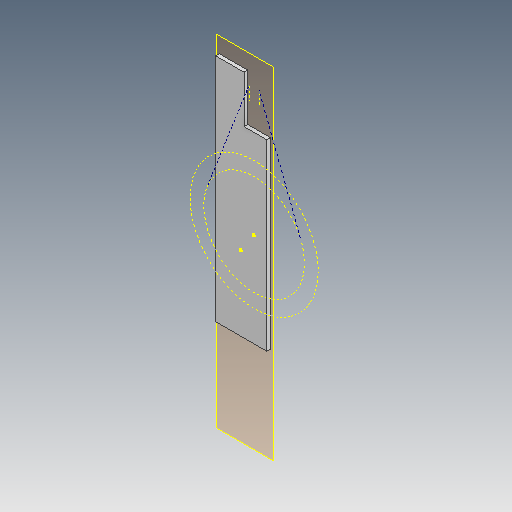
# Autodesk Inventor part: horizontal spool mount bottom
Saved by Autodesk Inventor 2020 (Build 240168000, 168)
## iProperties
Created: 2020-01-31
Part Number: horizontal spool mount bottom
Material: Generic
Document SubType Name: Modeling
Designer: ball
Density: 1 g/cm^3
Appearance: Default
Author: ball
Autodesk Inventor part; units mm, degrees
ref_plane "YZ Plane" through (0, 0, 0) normal (1, 0, 0) x (0, 1, 0)
ref_plane "XZ Plane" through (0, 0, 0) normal (0, 1, 0) x (-1, 0, 0)
ref_plane "XY Plane" through (0, 0, 0) normal (0, 0, 1) x (1, 0, 0)
ref_plane "Work Plane1" through (0, 0, 0) normal (0, 0, 1) x (1, 0, 0)
sketch "Sketch1" plane through (0, 0, 0) normal (0, 0, 1) x (1, 0, 0)
  line L0 (8.0002, 76.1) -> (3.2502, 76.1) construction
  line L1 (3.2502, 90.8) -> (3.2502, 103.5) construction
  line L2 (-17.75, 107.5) -> (-17.75, -107.5) construction
  line L3 (17.75, 107.5) -> (-17.75, 107.5) construction
  line L4 (1.9802, 107.5) -> (-17.75, 107.5)
  line L5 (-17.75, 107.5) -> (-17.75, 74.83)
  line L6 (-17.75, 74.83) -> (1.9802, 74.83)
  line L7 (1.9802, 74.83) -> (1.9802, 107.5)
  line L8 (-17.75, 74.83) -> (17.75, 74.83)
  line L9 (17.75, 74.83) -> (17.75, -52.17)
  line L10 (17.75, -52.17) -> (-17.75, -52.17)
  line L11 (-17.75, -52.17) -> (-17.75, 74.83)
  point P0 (0, 0)
  dimension "d1" = 1.27
  dimension "d2" = 1.27
  dimension "d5" = 127
  constraints: 24 end point, 4 horizontal, 4 parallel, 2 perpendicular, 2 point on line, 2 vertical, 7 other
  measures "d1" distance between parallel lines of L7 L1
  measures "d2" distance between parallel lines of L6 L0
  measures "d5" distance between parallel lines of L10 L8
extrude "Extrusion1" add sketch "Sketch1" along normal blind 2.54
sketch "Sketch2" plane through (0, 0, 2.54) normal (0, 0, 1) x (1, 0, 0)
  circle A0 centre (9.0001, 13.4819) radius 34.925 construction
  line L0 (12.3751, 101.9) -> (12.3751, 92.4) construction
  line L1 (5.6252, 92.4) -> (5.6252, 101.9) construction
  line L2 (-23.5916, 26.0332) -> (5.6252, 101.9) construction
  line L3 (41.5918, 26.0331) -> (12.3751, 101.9) construction
  point P0 (0, 0)
  constraints: 4 end point, 2 point on circle, 2 tangent
sketch "Sketch3" plane through (0, 0, 2.54) normal (0, 0, 1) x (1, 0, 0)
  circle A0 centre (9.0001, 13.4819) radius 44.45 construction
  point P0 (0, 0)
body "Solid1"
